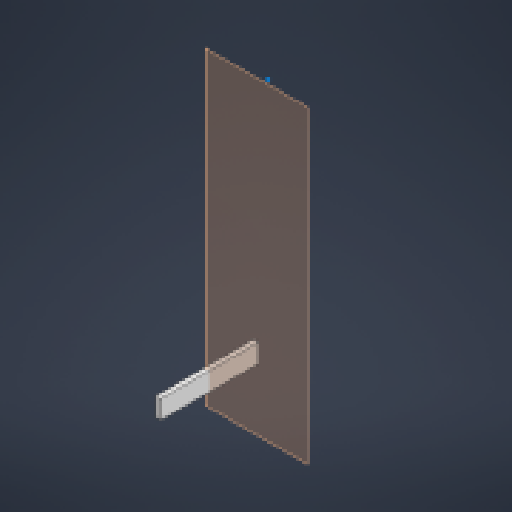
# Autodesk Inventor part: DoorFrameBase
Saved by Autodesk Inventor 2026.2 (Build 302298000, 298)
## iProperties
Created: 2026-03-06
Part Number: DoorFrameBase
Material: Generic
Document SubType Name: Modeling
Designer: brand
Density: 1 g/cm^3
Appearance: Default
Author: brand
Autodesk Inventor part; units mm, degrees
ref_plane "YZ Plane" through (0, 0, 0) normal (1, 0, 0) x (0, 1, 0)
ref_plane "XZ Plane" through (0, 0, 0) normal (0, 1, 0) x (-1, 0, 0)
ref_plane "XY Plane" through (0, 0, 0) normal (0, 0, 1) x (1, 0, 0)
ref_plane "Work Plane1" through (0, 0, 0) normal (0, 0, 1) x (1, 0, 0)
sketch "Sketch1" plane through (0, 0, 0) normal (0, 0, 1) x (1, 0, 0)
  line L0 (-351.028, -1081.278) -> (-389.128, -1081.278)
  line L1 (-389.128, -1081.278) -> (-389.128, -941.578)
  line L2 (-389.128, -941.578) -> (-351.028, -941.578)
  line L3 (-351.028, -941.578) -> (-351.028, -1081.278)
  line L4 (490.728, 1030.478) -> (-351.028, 1030.478) projected
  line L5 (-351.028, 1030.478) -> (-351.028, -1081.278) projected
  line L6 (-351.028, -1081.278) -> (490.728, -1081.278) projected
  line L7 (490.728, -1081.278) -> (490.728, 1030.478) projected
  line L8 (-312.928, -1043.178) -> (-312.928, 992.378) projected
  line L9 (-312.928, 992.378) -> (452.628, 992.378) projected
  line L10 (452.628, 992.378) -> (452.628, -1043.178) projected
  line L11 (452.628, -1043.178) -> (-312.928, -1043.178) projected
  point P0 (0, 0)
  point P1 (311.15, -1041.4)
  point P2 (349.25, -1079.5)
  dimension "d0" = 38.1
  dimension "d1" = 139.7
  constraints: 8 end point, 2 parallel, 1 horizontal, 1 perpendicular, 2 other
  measures "d0" distance of L1.end L2.end
  measures "d1" distance of L0.end L1.end
extrude "Extrusion1" add sketch "Sketch1" along normal mid plane 736.6 contours L0 L1 L2 L3
body "Solid1"
